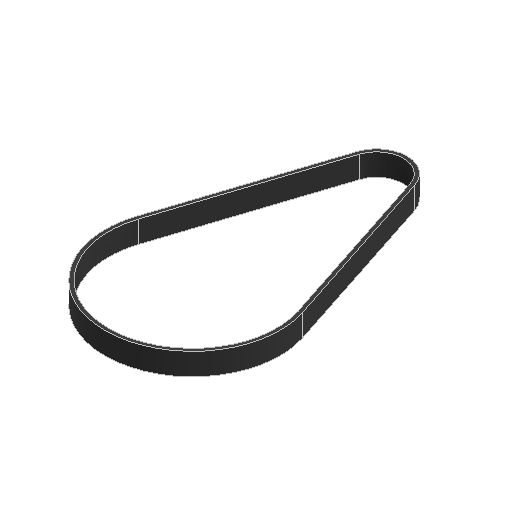
# Autodesk Inventor part: COTS_Optibelt_Omega_HTD3M_204T_6mm
Saved by Autodesk Inventor 2026.1 (Build 301233000, 233)
## iProperties
Created: 2024-07-27
Part Number: COTS_Optibelt_Omega_HTD3M_204T_6mm
Material: Generic
Document SubType Name: Modeling
Designer: User
Density: 1 g/cm^3
Appearance: Rubber - Black
Author: User
Autodesk Inventor part; units mm, degrees
ref_plane "YZ Plane" through (0, 0, 0) normal (1, 0, 0) x (0, 1, 0)
ref_plane "XZ Plane" through (0, 0, 0) normal (0, 1, 0) x (-1, 0, 0)
ref_plane "XY Plane" through (0, 0, 0) normal (0, 0, 1) x (1, 0, 0)
sketch "Sketch1" plane through (0, 0, 0) normal (0, 1, 0) x (-1, 0, 0)
  arc A0 (18.3066, 36.6819) -> (-24.9519, 36.6819) centre (-3.3227, 43.7344) ccw
  arc A1 (-10.2155, -8.5131) -> (3.5702, -8.5131) centre (-3.3227, -6.2656) ccw
  line L0 (-24.9519, 36.6819) -> (-10.2155, -8.5131)
  line L1 (18.3066, 36.6819) -> (3.5702, -8.5131)
  line L2 (-25.9027, 36.3719) -> (-11.1663, -8.8231)
  arc A2 (-11.1663, -8.8231) -> (4.5209, -8.8231) centre (-3.3227, -6.2656) ccw
  line L3 (4.5209, -8.8231) -> (19.2573, 36.3719)
  arc A3 (19.2573, 36.3719) -> (-25.9027, 36.3719) centre (-3.3227, 43.7344) ccw
  point P0 (0, 0)
  dimension "d0" = 45.5
  dimension "d1" = 14.5
  dimension "d2" = 50
  dimension "d3" = 1
  constraints: 8 end point, 8 point on circle, 4 centre point, 4 tangent, 1 vertical alignment, 3 other
  measures "d0" diameter of A0
  measures "d1" diameter of A1
  measures "d2" distance of A1.centre A0.centre
  measures "d3" radial gap between concentric circles of A0 A3
extrude "Extrusion1" add sketch "Sketch1" along normal blind 6
body "Solid1"
